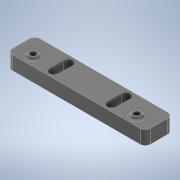
# Autodesk Inventor part: Rack support
Saved by Autodesk Inventor 2022 (Build 260153000, 153)
## iProperties
Created: 2022-03-06
Part Number: Rack support
Material: Genérico
Document SubType Name: Modeling
Designer: JK
Density: 1 g/cm^3
Appearance: Suave - Negro
Author: JK
Autodesk Inventor part; units mm, degrees
ref_plane "YZ Plane" through (0, 0, 0) normal (1, 0, 0) x (0, 1, 0)
ref_plane "XZ Plane" through (0, 0, 0) normal (0, 1, 0) x (-1, 0, 0)
ref_plane "XY Plane" through (0, 0, 0) normal (0, 0, 1) x (1, 0, 0)
sketch "Boceto1" plane through (0, 0, 0) normal (0, 1, 0) x (-1, 0, 0)
  line L0 (-40, 8) -> (40, 8)
  line L1 (40, 8) -> (40, -8)
  line L2 (40, -8) -> (-40, -8)
  line L3 (-40, -8) -> (-40, 8)
  line L4 (-40, 8) -> (40, -8) construction
  line L5 (40, 8) -> (-40, -8) construction
  circle A0 centre (-16.7, 4) radius 2.7
  circle A1 centre (-16.7, -4) radius 2.7
  circle A2 centre (16.7, 4) radius 2.7
  circle A3 centre (16.7, -4) radius 2.7
  line L6 (19.4, 4) -> (14, 4)
  line L7 (14, 4) -> (14, -4)
  line L8 (14, -4) -> (19.4, -4)
  line L9 (19.4, -4) -> (19.4, 4)
  line L10 (-14, 4) -> (-19.4, 4)
  line L11 (-19.4, 4) -> (-19.4, -4)
  line L12 (-19.4, -4) -> (-14, -4)
  line L13 (-14, -4) -> (-14, 4)
  point P0 (0, 0)
  point P1 (16.7, -4)
  point P2 (16.7, 4)
  point P3 (-16.7, -4)
  point P4 (-16.7, 4)
  point P5 (19.4, -4)
  point P6 (-14, -4)
  point P7 (-19.4, -4)
  point P8 (-19.4, 4)
  dimension "d2" = 5.4
  dimension "d0" = 80
  dimension "d1" = 16
  dimension "d3" = 4
  dimension "d4" = 8
  dimension "d5" = 23.3
  dimension "d35" = 23.3
  constraints: 28 end point, 7 midpoint, 6 parallel, 3 horizontal, 3 perpendicular, 3 vertical, 2 horizontal alignment, 1 centre point, 1 point on line, 1 tangent, 1 vertical alignment, 11 other
  measures "d0" distance of L1.end L2.end
  measures "d1" distance of L0.end L1.end
  measures "d3" vertical distance of point (0, 0) point (-16.7, 4)
  measures "d4" distance of L10.end L11.end
  measures "d5" distance from line of L3 point (-16.7, 4)
  measures "d35" distance from line of L1 point (16.7, -4)
extrude "Extrusión1" add sketch "Boceto1" along normal blind 8
fillet "Empalme2" radius 3 4 edges at (-40, 4, 8) (-40, 4, -8) (40, 4, 8) (40, 4, -8)
sketch "Boceto6" plane through (0, 8, 0) normal (0, 1, 0) x (1, 0, 0)
  circle A0 centre (-30, -3) radius 1.65
  circle A1 centre (30, -3) radius 1.65
  line L0 (37, 8) -> (-37, 8) projected
  line L1 (30, -3) -> (-30, -3)
  line L2 (-37, -8) -> (37, -8) projected
  point P0 (0, 0)
  dimension "d27" = 3.3
  dimension "d48" = 11
  dimension "d51" = 60
  dimension "d52" = 30
  constraints: 2 centre point, 2 end point, 1 equal radius, 1 horizontal alignment, 1 parallel
  measures "d27" diameter of A0
  measures "d48" distance from line of L0 L1.end
  measures "d51" distance of L1.start L1.end
  measures "d52" horizontal distance of point (0, 0) L1.start
extrude "Extrusión6" cut sketch "Boceto6" against normal through all
sketch "Boceto11" plane through (0, 0, 0) normal (0, -1, 0) x (1, 0, 0)
  circle A0 centre (-30, 3) radius 1.65 projected
  circle A1 centre (-30, 3) radius 2.9
  circle A2 centre (30, 3) radius 1.65 projected
  circle A3 centre (30, 3) radius 2.9
  line L0 (-32.9, 4.6743) -> (-30, 6.3486)
  line L1 (-30, 6.3486) -> (-27.1, 4.6743)
  line L2 (-27.1, 4.6743) -> (-27.1, 1.3257)
  line L3 (-27.1, 1.3257) -> (-30, -0.3486)
  line L4 (-30, -0.3486) -> (-32.9, 1.3257)
  line L5 (-32.9, 1.3257) -> (-32.9, 4.6743)
  line L6 (30, -0.3486) -> (27.1, 1.3257)
  line L7 (27.1, 1.3257) -> (27.1, 4.6743)
  line L8 (27.1, 4.6743) -> (30, 6.3486)
  line L9 (30, 6.3486) -> (32.9, 4.6743)
  line L10 (32.9, 4.6743) -> (32.9, 1.3257)
  line L11 (32.9, 1.3257) -> (30, -0.3486)
  point P0 (0, 0)
  dimension "d45" = 5.8
  constraints: 24 end point, 4 coincident, 2 centre point, 2 tangent, 2 vertical alignment, 1 equal radius, 26 other
  measures "d45" diameter of A3
extrude "Extrusión10" cut sketch "Boceto11" against normal blind 3 contours A0 | A1 | L2 L3 A1 | A1 L1 L2 | A1 L0 L1 | L3 L4 A1 | A1 L5 L0 | L4 L5 A1 | A2 | A3 | L10 L11 A3 | A3 L9 L10 | A3 L8 L9 | L11 L6 A3 | A3 L7 L8 | L6 L7 A3
sketch "Boceto12" plane through (0, 8, 0) normal (0, 1, 0) x (1, 0, 0)
  circle A0 centre (-30, -3) radius 1.65 projected
  circle A1 centre (-30, -3) radius 2.375
  circle A2 centre (30, -3) radius 1.65 projected
  circle A3 centre (30, -3) radius 2.375
  point P0 (0, 0)
  dimension "d53" = 4.75
  dimension "d54" = 4.75
  constraints: 2 centre point, 2 coincident
  measures "d53" diameter of A3
  measures "d54" diameter of A1
extrude "Extrusión11" add sketch "Boceto12" along normal blind 1.4
fillet "Empalme3" radius 1.4 2 edges at (-32.375, 8, 3) (27.625, 8, 3)
sketch "Boceto5" plane through (0, 0, 0) normal (0, -1, 0) x (1, 0, 0)
  circle A0 centre (-30, -4.1) radius 1.7 projected
  circle A1 centre (-30, -4.1) radius 2.875
  circle A2 centre (20, -4.1) radius 1.7 projected
  circle A3 centre (20, -4.1) radius 2.875
  line L0 (-33.3198, -4.1) -> (-31.6599, -1.225)
  line L1 (-31.6599, -1.225) -> (-28.3401, -1.225)
  line L2 (-28.3401, -1.225) -> (-26.6802, -4.1)
  line L3 (-26.6802, -4.1) -> (-28.3401, -6.975)
  line L4 (-28.3401, -6.975) -> (-31.6599, -6.975)
  line L5 (-31.6599, -6.975) -> (-33.3198, -4.1)
  line L6 (16.6802, -4.1) -> (18.3401, -1.225)
  line L7 (18.3401, -1.225) -> (21.6599, -1.225)
  line L8 (21.6599, -1.225) -> (23.3198, -4.1)
  line L9 (23.3198, -4.1) -> (21.6599, -6.975)
  line L10 (21.6599, -6.975) -> (18.3401, -6.975)
  line L11 (18.3401, -6.975) -> (16.6802, -4.1)
  point P0 (0, 0)
  dimension "d24" = 5.75
  constraints: 24 end point, 4 coincident, 2 centre point, 2 tangent, 1 equal radius, 1 horizontal, 1 horizontal alignment, 26 other
  measures "d24" diameter of A1
